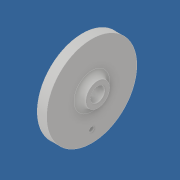
# Autodesk Inventor part: Brennerdeckel
Saved by Autodesk Inventor 2018 (Build 220112000, 112)
## iProperties
Created: 2018-10-23
Part Number: Brennerdeckel
Material: Generisch
Document SubType Name: Modeling
Designer: M.Knabel
Density: 1 g/cm^3
Appearance: Vorgabe
Author: M.Knabel
Autodesk Inventor part; units mm, degrees
ref_plane "YZ Plane" through (0, 0, 0) normal (1, 0, 0) x (0, 1, 0)
ref_plane "XZ Plane" through (0, 0, 0) normal (0, 1, 0) x (-1, 0, 0)
ref_plane "XY Plane" through (0, 0, 0) normal (0, 0, 1) x (1, 0, 0)
sketch "Skizze1" plane through (0, 0, 0) normal (0, 0, 1) x (1, 0, 0)
  line L0 (-1.3, 0) -> (7.8, 0) projected
  line L1 (0, -3.8) -> (0, 22.8) projected
  line L2 (0, 17.5) -> (0, 19)
  line L3 (0, 19) -> (4, 19)
  line L4 (4, 19) -> (4, 7.5)
  arc A0 (4, 7.5) -> (6.5, 5) centre (6.5, 7.5) ccw
  line L5 (6.5, 5) -> (6.5, 3)
  line L6 (6.5, 3) -> (2, 3)
  line L7 (2, 3) -> (2, 17.5)
  line L8 (0, 17.5) -> (2, 17.5)
  point P0 (0, 0)
  dimension "d0" = 38
  dimension "d1" = 35
  dimension "d2" = 6
  dimension "d3" = 2
  dimension "d4" = 4
  dimension "d5" = 6.5
  dimension "d6" = 2.5
  dimension "d7" = 10
  constraints: 14 end point, 4 perpendicular, 2 point on circle, 2 point on line, 1 centre point, 1 horizontal, 1 tangent, 1 vertical
  measures "d0" diameter of L3 L0
  measures "d1" diameter of L8 L0
  measures "d2" diameter of L6 L0
  measures "d3" distance between parallel lines of L1 L7
  measures "d4" distance between parallel lines of L1 L4
  measures "d5" distance between parallel lines of L1 L5
  measures "d6" radius of A0
  measures "d7" diameter of L5.start L0
revolve "Umdrehung1" add sketch "Skizze1" angle 360 about axis through (-10, 0, 0) along (1, 0, 0)
sketch "Skizze2" plane through (4, 0, 0) normal (1, 0, 0) x (0, 0, -1)
  line L0 (26.6, 0) -> (-26.6, 0) projected
  line L1 (0, -26.6) -> (0, 26.6) projected
  point P0 (0, 0)
  point P1 (14, 0)
  dimension "d9" = 14
  constraints: 1 point on line
  measures "d9" distance from line of point (14, 0) L1
hole "Bohrung1" at (4, 0, -14) direction (-1, 0, 0) diameter 2 end through all
